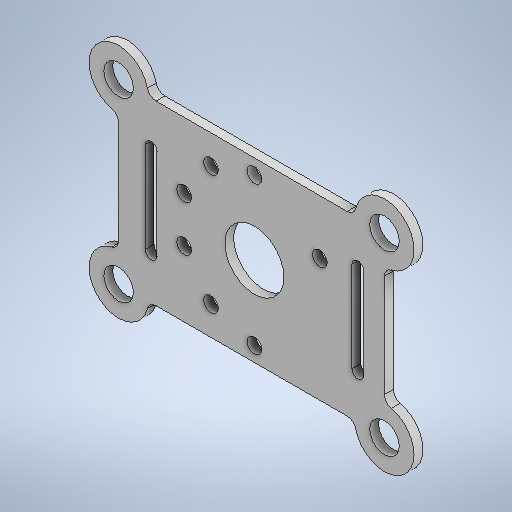
# Autodesk Inventor part: Desafio 3 - MASA - Inventor
Saved by Autodesk Inventor 2025.1 (Build 291241000, 241)
## iProperties
Created: 2025-05-20
Part Number: Desafio 3 - MASA - Inventor
Material: Generic
Document SubType Name: Modeling
Designer: Aluno
Density: 1 g/cm^3
Appearance: Default
Author: Aluno
Autodesk Inventor part; units mm, degrees
ref_plane "YZ Plane" through (0, 0, 0) normal (1, 0, 0) x (0, 1, 0)
ref_plane "XZ Plane" through (0, 0, 0) normal (0, 1, 0) x (-1, 0, 0)
ref_plane "XY Plane" through (0, 0, 0) normal (0, 0, 1) x (1, 0, 0)
sketch "Sketch1" plane through (0, 0, 0) normal (0, 0, 1) x (1, 0, 0)
  line L0 (-35.9682, 33.3635) -> (34.0318, 33.3635)
  line L1 (-45.9682, -16.6365) -> (-45.9682, 23.3635)
  circle A0 centre (-45.9682, 33.3635) radius 5
  circle A1 centre (44.0318, 33.3635) radius 5
  circle A2 centre (44.0318, -26.6365) radius 5
  circle A3 centre (-45.9682, -26.6365) radius 5
  arc A4 (-35.9682, 33.3635) -> (-45.9682, 23.3635) centre (-45.9682, 33.3635) ccw
  arc A5 (44.0318, 23.3635) -> (34.0318, 33.3635) centre (44.0318, 33.3635) ccw
  arc A6 (34.0318, -26.6365) -> (44.0318, -16.6365) centre (44.0318, -26.6365) ccw
  arc A7 (-45.9682, -16.6365) -> (-35.9682, -26.6365) centre (-45.9682, -26.6365) ccw
  line L2 (34.0318, -26.6365) -> (-35.9682, -26.6365)
  line L3 (44.0318, 23.3635) -> (44.0318, -16.6365)
  arc A8 (-33, 18.7271) -> (-37, 18.7271) centre (-35, 18.7271) ccw
  arc A9 (-37, -12) -> (-33, -12) centre (-35, -12) ccw
  arc A10 (37, 18.7271) -> (33, 18.7271) centre (35, 18.7271) ccw
  arc A11 (33, -12) -> (37, -12) centre (35, -12) ccw
  line L4 (-37, 18.7271) -> (-37, -12)
  line L5 (-33, -12) -> (-33, 18.7271)
  line L6 (33, 18.7271) -> (33, -12)
  line L7 (37, -12) -> (37, 18.7271)
  circle A12 centre (0, 3.3635) radius 10
  circle A13 centre (22.145, 14.9653) radius 2.5
  circle A14 centre (-14.6946, 23.589) radius 2.5
  circle A15 centre (-23.7764, 11.089) radius 2.5
  circle A16 centre (-23.7764, -4.3619) radius 2.5
  circle A17 centre (-14.6946, -16.8619) radius 2.5
  circle A18 centre (0, -21.6365) radius 2.5
  circle A19 centre (0, 28.3635) radius 2.5
  dimension "d22" = 242.35
  constraints: 20 centre point, 16 end point, 16 point on circle, 6 tangent, 4 coincident, 2 parallel, 1 horizontal, 1 perpendicular, 9 other
extrude "Extrusion1" add sketch "Sketch1" along normal blind 3
fillet "Fillet1" radius 3 8 edges at (-35.9682, 33.3635, 1.5) (44.0318, -16.6365, 1.5) (-45.9682, -16.6365, 1.5) (34.0318, 33.3635, 1.5) (34.0318, -26.6365, 1.5) (-45.9682, 23.3635, 1.5) (-35.9682, -26.6365, 1.5) (44.0318, 23.3635, 1.5)
body "Solid1"
